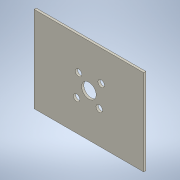
# Autodesk Inventor part: Gearbox Inner Mount
Saved by Autodesk Inventor 2022 (Build 260153000, 153)
## iProperties
Created: 2022-08-13
Part Number: Gearbox Inner Mount
Material: Steel, Galvanneal, A653 1010
Document SubType Name: Sheet Metal
Designer: Nick
Density: 7.86 g/cm^3
Sheet Metal Rule: STL A653 1010 Galvanneal .048 (19ga)
Appearance: Steel - Cast
Author: Nick
Autodesk Inventor part; units mm, degrees
ref_plane "YZ Plane" through (0, 0, 0) normal (1, 0, 0) x (0, 1, 0)
ref_plane "XZ Plane" through (0, 0, 0) normal (0, 1, 0) x (-1, 0, 0)
ref_plane "XY Plane" through (0, 0, 0) normal (0, 0, 1) x (1, 0, 0)
sketch "Sketch1" plane through (0, 0, 0) normal (0, 0, 1) x (1, 0, 0)
  line L0 (0, 0) -> (60, 0)
  line L1 (60, 0) -> (60, 47)
  line L2 (60, 47) -> (0, 47)
  line L3 (0, 47) -> (0, 0)
  circle A0 centre (30, 23.5) radius 4
  point P0 (60, 23.5)
  point P1 (30, 47)
  dimension "d0" = 60
  dimension "d1" = 47
  dimension "d2" = 8
  measures "d0" distance of L2.end L1.end
  measures "d1" distance of L1.end L0.end
  measures "d2" diameter of A0
extrude "Plate1" add sketch "Sketch1" along normal blind 1.2192
sketch "Sketch3" plane through (0, 0, 1.2192) normal (0, 0, 1) x (1, 0, 0)
  line L0 (23.2825, 16.7825) -> (36.7175, 30.2175) construction
  line L1 (24.3431, 29.1569) -> (35.6569, 17.8431) construction
  circle A0 centre (30, 23.5) radius 4 construction
  line L2 (30, 23.5) -> (30, 35.1596) construction
  point P0 (0, 0)
  dimension "d15" = 19
  dimension "d16" = 16
  dimension "d17" = 45
  constraints: 6 end point, 2 midpoint, 1 coincident, 1 perpendicular, 1 vertical
  measures "d15" distance of L0.start L0.end
  measures "d16" distance of L1.start L1.end
  measures "d17" angle of L0 L2
hole "Hole2" at (24.3431, 29.1569, 1.2192) at (35.6569, 17.8431, 1.2192) at (36.7175, 30.2175, 1.2192) at (23.2825, 16.7825, 1.2192) direction (0, 0, -1) diameter 3.6 end through all clearance for "Flat Head Machine Screw" size "M3" standard "Ansi Metric M Profile"
equation "\"d23\" = Thickness"
equation "\"d3\" = Thickness"
equation "\"BendReliefWidth\" = Thickness"
equation "\"BendReliefDepth\" = 0.5 * Thickness"
equation "\"CornerReliefSize\" = 3 * Thickness"
equation "\"MinimumRemnant\" = 2 * Thickness"
equation "\"TransitionRadius\" = BendRadius"
equation "\"JacobiRadiusSize\" = BendRadius"
equation "\"GapSize\" = 0.5 * Thickness"
equation "\"Thickness\" = 1.2192"
equation "\"BendRadius\" = 0.79375"
body "Solid1"
